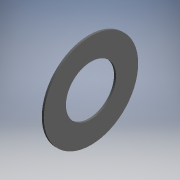
# Autodesk Inventor part: F624ZZ Shield1
Saved by Autodesk Inventor 2017.3 (Build 213256000, 256)
## iProperties
Part Number: F624ZZ Shield1
Material: Generic
Catalog Web Link: www.cadenas.de
Description: shielded_type_zz_zzs_S1-
Vendor: NSK_RB
Document SubType Name: Modeling
Designer: partserver
Manufacturer: NSK_RB
Mass: 0.0168691 g
Surface Area: 1.56758 cm^2
Volume: 0.0168691 cm^3
Density: 1 g/cm^3
Appearance: PSOLRGB-128-128-128
Category: PARTsolutions
Company: NSK_RB
Title: F624ZZ Shield1
Author: Cadenas PARTsolutions
PSOL_IDENT_0: {$CADENAS_DATA\23d-libs\nsk_rb\roller_bearings\deep_groove_bb\exstra_small_miniatur_bb\metric_design
PSOL_IDENT_1: _with_flange\shielded_type_zz_zzs_s1_1a.prj},186 {VTYP=3D},{NB=F624ZZ Shield1},{LINA=F624ZZ Shield1}
PSOL_IDENT_2: ,{NN=shielded_type_zz_zzs_S1},{DATE=16.07.2021 00:25:32},{GEOMDATE=04.01.2008 00:00:00},{VERSION=},{
PSOL_IDENT_3: LINEID=230},{WBVAR=},{WBNUMERIC=}  {NB=F624ZZ Shield1},{LINA=F624ZZ Shield1},{KT=DUMMY},{IDNR=},{STA
PSOL_IDENT_4: N=},{ORDER=F624ZZ},{SD=4.0},{X=4.0},{D=13},{DD=13},{DD1=0.0},{D2=15.0},{DD2=15.0},{B=0.0},{B1=5.0},{
PSOL_IDENT_5: CC1=0.0},{C2=1.0},{CC2=1.0},{R=0.00},{R1=0.20},{DI1=6.95},{DI2=6.00},{SDE1=10.45},{SDE2=11.30},{CR1=
PSOL_IDENT_6: 1300},{COR1=485},{CR2=133},{COR2=49.0},{LG=40000},{LO=48000},{DA=0.0},{DB=6.0},{RA=0.00},{RB=0.20},{
PSOL_IDENT_7: MASS=3.53},{SC=1}
NB: F624ZZ Shield1
NN: shielded_type_zz_zzs_S1
NBSYN: $ORDER. Shield1
LINA: F624ZZ Shield1
CATALOG: NSK Rolling Bearing
ORDER: F624ZZ
SD: 4
X: 4
D: 13
DD: 13
DD1: 0
D2: 15
DD2: 15
B: 0
B1: 5
CC1: 0
C2: 1
CC2: 1
R: 0
R1: 0.2
DI1: 6.95
DI2: 6
SDE1: 10.45
SDE2: 11.3
CR1: 1300
COR1: 485
CR2: 133
COR2: 49
LG: 40000
LO: 48000
DA: 0
DB: 6
RA: 0
RB: 0.2
MASS: 3.53
SC: 1
SUPPLIER: NSK_RB
ARTICLENO: F624ZZ Shield1
BOMINFO: F624ZZ Shield1
CREATOR: CADENAS GmbH
Autodesk Inventor part; units mm, degrees
sketch "Sketch_1" plane through (0, 0, 0) normal (0, 0, 1) x (1, 0, 0)
  line L0 (0.5468, 0) -> (0.3125, 0)
  line L1 (0.3125, 3) -> (0.5468, 3)
  line L2 (0.5468, 3) -> (0.5468, 5.65)
  line L3 (0.5468, 5.65) -> (0.3125, 5.65)
  line L4 (0.3125, 5.65) -> (0.3125, 3)
  constraints: 10 end point
revolve "Revolution1" add sketch "Sketch_1" angle 360 about axis through (0.5468, 0, 0) along (1, 0, 0)
ref_plane "ip_st_1_XY" through (0.3125, 0, 0) normal (-1, 0, 0) x (0, 0, -1)
ref_plane "ip_st_1_YZ" through (0.3125, 0, 0) normal (0, 0, -1) x (0, -1, 0)
ref_plane "ip_st_1_ZX" through (0.3125, 0, 0) normal (0, -1, 0) x (-1, 0, 0)
body "Solid1"
